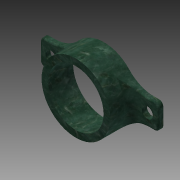
# Autodesk Inventor part: Big Bearing Mount
Saved by Autodesk Inventor 2014 (Build 180170000, 170)
## iProperties
Created: 2015-02-12
Part Number: Big Bearing Mount
Material: Generic
Document SubType Name: Modeling
Designer: Spooner
Density: 1 g/cm^3
Appearance: Green Polished
Author: Spooner
Autodesk Inventor part; units mm, degrees
ref_plane "YZ Plane" through (0, 0, 0) normal (1, 0, 0) x (0, 1, 0)
ref_plane "XZ Plane" through (0, 0, 0) normal (0, 1, 0) x (-1, 0, 0)
ref_plane "XY Plane" through (0, 0, 0) normal (0, 0, 1) x (1, 0, 0)
ref_plane "Work Plane1" through (0, 0, 0) normal (0, 0, 1) x (1, 0, 0)
sketch "Sketch1" plane through (0, 0, 0) normal (0, 0, 1) x (1, 0, 0)
  circle A0 centre (0, 0) radius 23.495 projected
  circle A1 centre (0, 0) radius 23.749
  circle A2 centre (0, 0) radius 26.289
  point P0 (0, 0)
  dimension "d0" = 0.254
  dimension "d1" = 2.54
  constraints: 2 centre point, 2 coincident
  measures "d0" radial gap between concentric circles of A0 A1
  measures "d1" radial gap between concentric circles of A1 A2
ref_plane "Work Plane2" through (-23.495, -23.495, -13.97) normal (0, 0, -1) x (0, 1, 0)
extrude "Extrusion1" add sketch "Sketch1" against normal up to surface (13.97 mm away) contours A2
sketch "Sketch2" plane through (0, 0, 0) normal (0, 0, 1) x (1, 0, 0)
  circle A0 centre (0, 0) radius 23.749 projected
  circle A1 centre (0, 0) radius 26.289 projected
  circle A2 centre (0, 0) radius 21.209
  dimension "d4" = 2.54
  constraints: 1 centre point, 1 coincident
  measures "d4" radial gap between concentric circles of A0 A2
sketch "Sketch3" plane through (0, 0, -13.97) normal (0, 0, -1) x (-1, 0, 0)
  circle A0 centre (0, 0) radius 23.749 projected
  circle A1 centre (0, 0) radius 26.289 projected
  line L0 (-24.5028, 9.525) -> (-45.339, 9.525)
  line L1 (-45.339, 9.525) -> (-45.339, -9.525)
  line L2 (-45.339, -9.525) -> (-24.5028, -9.525)
  line L3 (24.5028, 9.525) -> (45.339, 9.525)
  line L4 (45.339, 9.525) -> (45.339, -9.525)
  line L5 (45.339, -9.525) -> (24.5028, -9.525)
  dimension "d7" = 19.05
  dimension "d8" = 19.05
  dimension "d9" = 19.05
  dimension "d10" = 9.525
  constraints: 12 end point, 4 point on circle, 3 parallel, 2 horizontal alignment, 2 perpendicular, 1 horizontal
  measures "d7" distance of L0.end L1.end
  measures "d8" distance edge to line of A1 L1
  measures "d9" distance edge to line of A1 L4
  measures "d10" distance from line of A0.centre L0
extrude "Extrusion3" add sketch "Sketch3" against normal blind 3.81 contours A1 L3 L4 L5 | A1 L2 L1 L0
fillet "Fillet1" radius 25.4 4 edges at (24.5028, 9.525, -12.065) (-24.5028, 9.525, -12.065) (24.5028, -9.525, -12.065) (-24.5028, -9.525, -12.065)
fillet "Fillet2" radius 6.35 7 edges at (-22.3248, -13.8822, -10.16) (-26.289, 0, -10.16) (-22.3248, 13.8822, -10.16) (22.3248, -13.8822, -10.16) (25.8386, -4.8455, -10.16) (25.8386, 4.8455, -10.16) (22.3248, 13.8822, -10.16)
fillet "Fillet3" radius 3.175 4 edges at (45.339, -9.525, -12.065) (45.339, 9.525, -12.065) (-45.339, -9.525, -12.065) (-45.339, 9.525, -12.065)
sketch "Sketch4" plane through (0, 0, -10.16) normal (0, 0, 1) x (1, 0, 0)
  line L0 (-45.339, 6.35) -> (-45.339, -6.35) projected
  arc A0 (-30.8785, 10.5747) -> (-30.8785, -10.5747) centre (0, 0) ccw projected
  arc A1 (45.339, 6.35) -> (42.164, 9.525) centre (42.164, 6.35) ccw projected
  line L1 (42.164, 9.525) -> (38.1051, 9.525) projected
  arc A2 (30.8785, 10.5747) -> (38.1051, 9.525) centre (38.1051, 34.925) ccw projected
  arc A3 (30.8785, -10.5747) -> (30.8785, 10.5747) centre (0, 0) ccw projected
  arc A4 (38.1051, -9.525) -> (30.8785, -10.5747) centre (38.1051, -34.925) ccw projected
  line L2 (38.1051, -9.525) -> (42.164, -9.525) projected
  arc A5 (42.164, -9.525) -> (45.339, -6.35) centre (42.164, -6.35) ccw projected
  line L3 (45.339, -6.35) -> (45.339, 6.35) projected
  circle A6 centre (-36.957, 0) radius 4.191
  circle A7 centre (36.957, 0) radius 4.191
  dimension "d16" = 8.382
  dimension "d17" = 8.382
  dimension "d18" = 8.382
  constraints: 2 centre point, 2 horizontal alignment, 1 equal radius
  measures "d16" diameter of A6
  measures "d17" distance from line of A6.centre L0
  measures "d18" distance from line of A7.centre L3
extrude "Extrusion4" cut sketch "Sketch4" against normal through all contours A6 | A7
extrude "Extrusion5" add sketch "Sketch2" along normal blind 5.08 contours A1
sketch "Sketch5" plane through (0, 0, 5.08) normal (0, 0, 1) x (1, 0, 0)
  circle A0 centre (0, 0) radius 23.749 projected
  circle A1 centre (0, 0) radius 26.289 projected
  circle A2 centre (0, 0) radius 21.209
  dimension "d23" = 2.54
  constraints: 1 centre point, 1 coincident
  measures "d23" radial gap between concentric circles of A0 A2
extrude "Extrusion6" add sketch "Sketch5" along normal blind 2.54 contours A0 | A1
fillet "Fillet4" radius 1.27 22 edges at (-34.4539, -9.7888, -10.16) (-40.1345, -9.525, -10.16) (-44.4091, -8.5951, -10.16) (-45.339, 0, -10.16) (-44.4091, 8.5951, -10.16) (-40.1345, 9.525, -10.16) (-34.4539, 9.7888, -10.16) (-23.3928, 14.2197, -7.3623) (-29.8848, 10.892, -10.1054) (-29.8848, -10.892, -10.1054) (-23.3928, -14.2197, -7.3623) (23.3928, -14.2197, -7.3623) (29.8848, -10.892, -10.1054) (40.1345, -9.525, -10.16) (44.4091, -8.5951, -10.16) (45.339, 0, -10.16) (44.4091, 8.5951, -10.16) (40.1345, 9.525, -10.16) (34.4539, 9.7888, -10.16) (29.8848, 10.892, -10.1054) (23.3928, 14.2197, -7.3623) (34.4539, -9.7888, -10.16)
equation "\"d9\" = d8"
equation "\"d10\" = 0.5 * d7"
equation "\"d18\" = d17"
body "Solid1"
